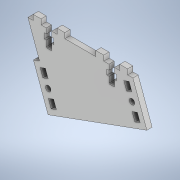
# Autodesk Inventor part: tc_support_front
Saved by Autodesk Inventor 2020.1 (Build 241239000, 239)
## iProperties
Created: 2019-07-16
Part Number: tc_support_front
Material: Acier inoxydable
Document SubType Name: Modeling
Designer: Thibault
Density: 8 g/cm^3
Appearance: Semi-poli
anchor_dist_b: 36.000 mm
anchor_dist_a: 2,000 mm
anchor_dist_top_a: 8.000 mm
tilt_angle: 20,00 deg
tc_plates_dist: 34,000 mm
Author: Thibault
Autodesk Inventor part; units mm, degrees
ref_plane "YZ Plane" through (0, 0, 0) normal (1, 0, 0) x (0, 1, 0)
ref_plane "XZ Plane" through (0, 0, 0) normal (0, 1, 0) x (-1, 0, 0)
ref_plane "XY Plane" through (0, 0, 0) normal (0, 0, 1) x (1, 0, 0)
sketch "Anchor (screw side)" plane through (0, 0, 0) normal (0, 0, 1) x (1, 0, 0)
  circle A0 centre (93.8994, 50.3042) radius 1.05
  line L0 (90.8494, 51.3542) -> (87.7494, 51.3542)
  line L1 (87.7494, 51.3542) -> (87.7494, 49.2542)
  line L2 (87.7494, 49.2542) -> (90.8494, 49.2542)
  line L3 (90.8494, 49.2542) -> (90.8494, 51.3542)
  line L4 (100.0494, 51.3542) -> (96.9494, 51.3542)
  line L5 (96.9494, 51.3542) -> (96.9494, 49.2542)
  line L6 (96.9494, 49.2542) -> (100.0494, 49.2542)
  line L7 (100.0494, 49.2542) -> (100.0494, 51.3542)
  line L8 (90.8494, 51.3542) -> (96.9494, 49.2542) construction
  line L9 (96.9494, 51.3542) -> (90.8494, 49.2542) construction
  line L10 (85.7494, 53.3542) -> (102.0494, 53.3542) construction
  line L11 (102.0494, 53.3542) -> (102.0494, 47.2542) construction
  line L12 (102.0494, 47.2542) -> (85.7494, 47.2542) construction
  line L13 (85.7494, 47.2542) -> (85.7494, 53.3542) construction
  point P0 (103.5798, 50.1132)
  dimension "d27" = 2.1
  dimension "d28" = 3.1
  dimension "d29" = 2.1
  dimension "slot_distance" = 6.1
  dimension "d34" = 2
  dimension "d35_1" = 2
  dimension "d36_1" = 2
  dimension "d37" = 2
  measures "d27" diameter of A0
  measures "d28" distance of L2.end L1.end
  measures "d29" distance of L1.end L0.end
  measures "slot_distance" distance between parallel lines of L5 L3
  measures "d34" distance between parallel lines of L0 L10
  measures "d35_1" distance between parallel lines of L12 L2
  measures "d36_1" distance between parallel lines of L11 L7
  measures "d37" distance between parallel lines of L13 L1
sketch "Anchor (nut side)" plane through (0, 0, 0) normal (0, 0, 1) x (1, 0, 0)
  line L0 (11.1, 0) -> (9.1, 0)
  line L1 (9.1, 0) -> (9.1, -2)
  line L2 (9.1, -2) -> (9.9, -2)
  line L3 (9.9, -2) -> (9.9, -4)
  line L4 (6.2, -4) -> (6.2, -2)
  line L5 (6.2, -2) -> (7, -2)
  line L6 (7, -2) -> (7, 0)
  line L7 (7, 0) -> (5, 0)
  line L8 (2, 0) -> (2, 2)
  line L9 (2, 0) -> (3, 0) construction
  line L10 (2, 2) -> (5, 2)
  line L11 (5, 2) -> (5, 0)
  line L12 (11.1, 0) -> (11.1, 2)
  line L13 (11.1, 2) -> (14.1, 2)
  line L14 (14.1, 2) -> (14.1, 0)
  line L15 (0, 0) -> (2, 0)
  line L16 (14.1, 0) -> (16.1, 0)
  line L17 (6.2, -4) -> (7, -4)
  line L18 (9.9, -4) -> (9.1, -4)
  line L19 (7, -4) -> (7, -6.25)
  line L20 (9.1, -4) -> (9.1, -6.25)
  line L21 (7.25, -6.5) -> (8.05, -6.5)
  arc A0 (7, -6.25) -> (7.25, -6.5) centre (7.25, -6.25) ccw
  arc A1 (8.85, -6.5) -> (9.1, -6.25) centre (8.85, -6.25) ccw
  line L22 (8.05, -6.5) -> (8.85, -6.5)
  line L23 (8.05, -3.8983) -> (8.05, -9.959) construction
  point P0 (9.1321, -0.6227)
  point P1 (7, -6.5)
  point P2 (9.1, -6.5)
  dimension "d3" = 2
  dimension "d7" = 6.1
  dimension "d10" = 2
  dimension "d11" = 2
  dimension "d12" = 0.8
  dimension "d13" = 2
  dimension "d14" = 0.8
  dimension "d15" = 2.1
  dimension "d18" = 2
  dimension "d19" = 0.8
  dimension "d20" = 0.8
  dimension "d21" = 2.5
  dimension "d22" = 2.5
  dimension "d23" = 2.1
  dimension "d38" = 2
  dimension "d39" = 0.25
  dimension "d120" = 3
  measures "d3" distance of L15.start L8.start
  measures "d7" distance of L7.end L0.start
  measures "d10" distance of L0.start L0.end
  measures "d11" distance of L0.end L1.end
  measures "d12" distance of L1.end L2.end
  measures "d13" distance of L2.end L3.end
  measures "d14" distance of L4.end L5.end
  measures "d15" distance of L6.end L0.end
  measures "d18" distance of L14.end L16.end
  measures "d19" distance of L4.start L17.end
  measures "d20" distance of L3.end L18.end
  measures "d21" distance of L17.end point (7, -6.5)
  measures "d22" distance of L18.end point (9.1, -6.5)
  measures "d23" distance of L17.end L18.end
  measures "d38" distance between parallel lines of L15 L10
  measures "d39" radius of A0
  measures "d120" distance of L8.end L10.end
derived "shared_parameters.ipt"
sketch "Esquisse1" plane through (0, 0, 0) normal (0, 0, 1) x (1, 0, 0)
  line L0 (82.7538, -31.3802) -> (77.4343, -16.7648)
  line L1 (82.7538, -31.3802) -> (47.3888, -44.252)
  line L2 (-2.0657, -1.8526) -> (7.9343, -1.7975) construction
  line L3 (41.8139, -28.935) -> (37.3843, -16.7648)
  line L4 (53.4843, -16.7648) -> (61.3343, -16.7648)
  line L5 (39.4972, -29.7782) -> (45.0722, -45.0952)
  line L6 (39.4972, -29.7782) -> (41.8139, -28.935)
  line L7 (47.3888, -44.252) -> (47.3888, -44.252)
  line L8 (45.0722, -45.0952) -> (47.3888, -44.252)
  circle A0 centre (77.1003, -24.7648) radius 1.05
  line L9 (77.1568, -27.99) -> (78.217, -30.9031)
  line L10 (78.217, -30.9031) -> (80.1904, -30.1848)
  line L11 (80.1904, -30.1848) -> (79.1301, -27.2718)
  line L12 (79.1301, -27.2718) -> (77.1568, -27.99)
  line L13 (74.0102, -19.3448) -> (75.0705, -22.2579)
  line L14 (75.0705, -22.2579) -> (77.0438, -21.5396)
  line L15 (77.0438, -21.5396) -> (75.9836, -18.6266)
  line L16 (75.9836, -18.6266) -> (74.0102, -19.3448)
  line L17 (77.1568, -27.99) -> (77.0438, -21.5396) construction
  line L18 (75.0705, -22.2579) -> (79.1301, -27.2718) construction
  line L19 (77.0217, -33.4665) -> (71.4468, -18.1495) construction
  line L20 (71.4468, -18.1495) -> (77.1789, -16.0632) construction
  line L21 (77.1789, -16.0632) -> (82.7538, -31.3802) construction
  line L22 (82.7538, -31.3802) -> (77.0217, -33.4665) construction
  circle A1 centre (45.1508, -36.3935) radius 1.05
  line L23 (45.0943, -33.1683) -> (44.034, -30.2553)
  line L24 (44.034, -30.2553) -> (42.0606, -30.9735)
  line L25 (42.0606, -30.9735) -> (43.1209, -33.8866)
  line L26 (43.1209, -33.8866) -> (45.0943, -33.1683)
  line L27 (48.2409, -41.8135) -> (47.1806, -38.9004)
  line L28 (47.1806, -38.9004) -> (45.2072, -39.6187)
  line L29 (45.2072, -39.6187) -> (46.2675, -42.5317)
  line L30 (46.2675, -42.5317) -> (48.2409, -41.8135)
  line L31 (45.0943, -33.1683) -> (45.2072, -39.6187) construction
  line L32 (47.1806, -38.9004) -> (43.1209, -33.8866) construction
  line L33 (45.2293, -27.6918) -> (50.8043, -43.0088) construction
  line L34 (50.8043, -43.0088) -> (45.0722, -45.0952) construction
  line L35 (45.0722, -45.0952) -> (39.4972, -29.7782) construction
  line L36 (39.4972, -29.7782) -> (45.2293, -27.6918) construction
  line L37 (48.4843, -16.7648) -> (46.4843, -16.7648)
  line L38 (46.4843, -16.7648) -> (46.4843, -18.7648)
  line L39 (46.4843, -18.7648) -> (47.2843, -18.7648)
  line L40 (47.2843, -18.7648) -> (47.2843, -20.7648)
  line L41 (43.5843, -20.7648) -> (43.5843, -18.7648)
  line L42 (43.5843, -18.7648) -> (44.3843, -18.7648)
  line L43 (44.3843, -18.7648) -> (44.3843, -16.7648)
  line L44 (44.3843, -16.7648) -> (42.3843, -16.7648)
  line L45 (39.3843, -16.7648) -> (39.3843, -14.7648)
  line L46 (39.3843, -16.7648) -> (40.3843, -16.7648) construction
  line L47 (39.3843, -14.7648) -> (42.3843, -14.7648)
  line L48 (42.3843, -14.7648) -> (42.3843, -16.7648)
  line L49 (48.4843, -16.7648) -> (48.4843, -14.7648)
  line L50 (48.4843, -14.7648) -> (51.4843, -14.7648)
  line L51 (51.4843, -14.7648) -> (51.4843, -16.7648)
  line L52 (37.3843, -16.7648) -> (39.3843, -16.7648)
  line L53 (51.4843, -16.7648) -> (53.4843, -16.7648)
  line L54 (43.5843, -20.7648) -> (44.3843, -20.7648)
  line L55 (47.2843, -20.7648) -> (46.4843, -20.7648)
  line L56 (44.3843, -20.7648) -> (44.3843, -23.0148)
  line L57 (46.4843, -20.7648) -> (46.4843, -23.0148)
  line L58 (44.6343, -23.2648) -> (45.4343, -23.2648)
  arc A2 (44.3843, -23.0148) -> (44.6343, -23.2648) centre (44.6343, -23.0148) ccw
  arc A3 (46.2343, -23.2648) -> (46.4843, -23.0148) centre (46.2343, -23.0148) ccw
  line L59 (45.4343, -23.2648) -> (46.2343, -23.2648)
  line L60 (45.4343, -20.6631) -> (45.4343, -26.7238) construction
  line L61 (72.4343, -16.7648) -> (70.4343, -16.7648)
  line L62 (70.4343, -16.7648) -> (70.4343, -18.7648)
  line L63 (70.4343, -18.7648) -> (71.2343, -18.7648)
  line L64 (71.2343, -18.7648) -> (71.2343, -20.7648)
  line L65 (67.5343, -20.7648) -> (67.5343, -18.7648)
  line L66 (67.5343, -18.7648) -> (68.3343, -18.7648)
  line L67 (68.3343, -18.7648) -> (68.3343, -16.7648)
  line L68 (68.3343, -16.7648) -> (66.3343, -16.7648)
  line L69 (63.3343, -16.7648) -> (63.3343, -14.7648)
  line L70 (63.3343, -16.7648) -> (64.3343, -16.7648) construction
  line L71 (63.3343, -14.7648) -> (66.3343, -14.7648)
  line L72 (66.3343, -14.7648) -> (66.3343, -16.7648)
  line L73 (72.4343, -16.7648) -> (72.4343, -14.7648)
  line L74 (72.4343, -14.7648) -> (75.4343, -14.7648)
  line L75 (75.4343, -14.7648) -> (75.4343, -16.7648)
  line L76 (61.3343, -16.7648) -> (63.3343, -16.7648)
  line L77 (75.4343, -16.7648) -> (77.4343, -16.7648)
  line L78 (67.5343, -20.7648) -> (68.3343, -20.7648)
  line L79 (71.2343, -20.7648) -> (70.4343, -20.7648)
  line L80 (68.3343, -20.7648) -> (68.3343, -23.0148)
  line L81 (70.4343, -20.7648) -> (70.4343, -23.0148)
  line L82 (68.5843, -23.2648) -> (69.3843, -23.2648)
  arc A4 (68.3343, -23.0148) -> (68.5843, -23.2648) centre (68.5843, -23.0148) ccw
  arc A5 (70.1843, -23.2648) -> (70.4343, -23.0148) centre (70.1843, -23.0148) ccw
  line L83 (69.3843, -23.2648) -> (70.1843, -23.2648)
  line L84 (69.3843, -20.6631) -> (69.3843, -26.7238) construction
  point P0 (77.1003, -24.7648)
  point P1 (45.1508, -36.3935)
  dimension "d44" = 2
  dimension "d45" = 0.4653
  dimension "d55" = 40.05
  dimension "tc_plates_dist" = 34
  constraints: 18 end point, 3 horizontal, 2 perpendicular, 2 point on line, 1 collinear, 1 parallel, 14 other
  measures "d55" distance of L3.end L0.end
  measures "tc_plates_dist" distance of point (45.151, -36.394) point (77.1, -24.765)
extrude "Extrusion1" add sketch "Esquisse1" along normal blind 2
equation "\"d55\" = tc_base_back_width"
equation "\"d35\" = sheet_thickness"
equation "\"tc_base_back_width\" = 40.05"
equation "\"sheet_thickness\" = 2"
